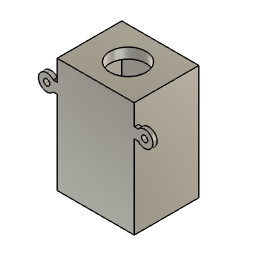
battery holder_ (Autodesk Fusion 360 design; units mm, degrees)
Autodesk Fusion 360 part; units mm, degrees
note: some values were not read from the file. Set by a fixed rule: which sketch regions a step uses.
sketch "Sketch1" plane through (0, 0, 0) normal (0, 0, 1) x (1, 0, 0)
  line L0 (0, 50) -> (37, 50)
  line L1 (37, 50) -> (37, 19)
  line L2 (37, 19) -> (0, 19)
  line L3 (0, 19) -> (0, 50)
  line L4 (3, 22) -> (3, 47)
  line L5 (3, 47) -> (34, 47)
  line L6 (34, 47) -> (34, 22)
  line L7 (34, 22) -> (3, 22)
  dimension "d1" = 37
  dimension "d2" = 31
  dimension "d3" = 3
  constraint horizontal L0
  constraint vertical L1
  constraint horizontal L2
  constraint vertical L3
  measures "d1" distance of L0.start L0.end
  measures "d2" distance of L0.start L2.end
extrude "Extrude1" add sketch "Sketch1" along normal blind 55
sketch "Sketch2" plane through (0, 0, 55) normal (0, 0, 1) x (-1, 0, 0)
  line L0 (-34, -47) -> (-34, -22)
  line L1 (-34, -22) -> (-3, -22)
  line L2 (-3, -22) -> (-3, -47)
  line L3 (-3, -47) -> (-34, -47)
  line L4 (0, -19) -> (-37, -19)
  line L5 (-37, -19) -> (-37, -50)
  line L6 (-37, -50) -> (0, -50)
  line L7 (0, -50) -> (0, -19)
  line L8 (0, -50) -> (-37, -50)
  line L9 (-37, -50) -> (-37, -19)
  line L10 (-37, -19) -> (0, -19)
  line L11 (0, -19) -> (0, -50)
  circle A0 centre (-18.5, -34.5) radius 8.6861
  constraint horizontal L8
  constraint vertical L9
  constraint horizontal L10
  constraint vertical L11
  constraint coincident L4.end L5.start
  constraint coincident L6.end L7.start
extrude "Extrude2" add sketch "Sketch2" against normal blind 5 contours L0 L1 L2 L3 | L4 L5 L6 L7 L8 L9 L10 L11
sketch "Sketch3" plane through (0, 19, 0) normal (0, -1, 0) x (1, 0, 0)
  line L0 (0, 55) -> (0, 0)
  line L1 (0, 0) -> (37, 0)
  line L2 (37, 0) -> (37, 55)
  line L3 (37, 55) -> (0, 55)
  line L4 (0, 40) -> (-5, 40)
  line L5 (-5, 40) -> (-5, 45)
  line L6 (-5, 45) -> (0, 45)
  line L7 (0, 45) -> (0, 40)
  line L8 (37, 40) -> (42, 40)
  line L9 (42, 40) -> (42, 45)
  line L10 (42, 45) -> (37, 45)
  circle A0 centre (-5, 42.5) radius 1.5
  circle A1 centre (-5, 42.5) radius 4
  circle A2 centre (42, 42.5) radius 1.5
  circle A3 centre (42, 42.5) radius 4
  line L11 (35, 40) -> (38, 40)
  line L12 (38, 40) -> (38, 45)
  line L13 (38, 45) -> (35, 45)
  line L14 (1.6164, 40) -> (-1, 40)
  line L15 (-1, 40) -> (-1, 45)
  line L16 (-1, 45) -> (1.6164, 45)
  line L17 (35, 40) -> (35, 45)
  line L18 (1.6164, 40) -> (1.6164, 45)
  dimension "d9" = 5
  dimension "d10" = 3
  dimension "d11" = 2.5
  dimension "d12" = 3
  dimension "d13" = 2.5
  constraint horizontal L4
  constraint vertical L5
  constraint horizontal L6
  constraint vertical L7
  constraint coincident L0 L4.start
  constraint horizontal L8
  constraint vertical L9
  constraint horizontal L10
  constraint coincident L2 L8.start
  constraint midpoint L5 A0.centre
  constraint midpoint L9 A2.centre
  constraint horizontal L11
  constraint vertical L12
  constraint horizontal L13
  constraint coincident L10 L12.end
  constraint horizontal L14
  constraint vertical L15
  constraint horizontal L16
  constraint coincident L6 L15.end
  constraint perpendicular L13 L17
  constraint perpendicular L16 L18
  measures "d9" distance of L8.start L8.end
  measures "d10" diameter of A0
  measures "d12" diameter of A2
extrude "Extrude3" add sketch "Sketch3" against normal blind 2 contours L0 L7 L14 L16 L18 | L0 L4 L6 L7 L14 L15 L16 | L6 A1 L15 | L2 L8 L10 L11 L12 L13 | L2 L11 L13 L17 | L4 A1 L15 | L4 L5 L6 A0 A1 | L4 L5 L6 A0 A1 | L10 A3 L12 | L8 A3 L12 | L8 L9 L10 A2 A3 | L8 L9 L10 A2 A3
